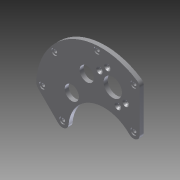
# Autodesk Inventor part: back plate
Saved by Autodesk Inventor 2012 (Build 160160000, 160)
## iProperties
Created: 2012-02-08
Part Number: back plate
Material: Default
Document SubType Name: Modeling
Designer: Antonella Wilby
Density: 1 g/cm^3
Author: Antonella Wilby
Autodesk Inventor part; units mm, degrees
ref_plane "YZ Plane" through (0, 0, 0) normal (1, 0, 0) x (0, 1, 0)
ref_plane "XZ Plane" through (0, 0, 0) normal (0, 1, 0) x (-1, 0, 0)
ref_plane "XY Plane" through (0, 0, 0) normal (0, 0, 1) x (1, 0, 0)
sketch "Sketch1" plane through (0, 0, 0) normal (0, 0, 1) x (1, 0, 0)
  line L0 (-166.2465, 0) -> (95.1399, 0) projected
  line L1 (0, -97.3562) -> (0, 206.312) projected
  circle A0 centre (0, 0) radius 53.975 construction
  arc A1 (39.2886, 39.2886) -> (-55.3511, 4.8426) centre (0, 0) ccw
  line L2 (0, 0) -> (-102.554, 102.554) construction
  circle A2 centre (-50.2894, 50.2894) radius 11.1506
  circle A3 centre (-50.2894, 50.2894) radius 13.335 construction
  circle A4 centre (-50.2894, 50.2894) radius 39.37 construction
  circle A5 centre (-26.9875, 87.3943) radius 11.1506
  circle A6 centre (-26.9875, 87.3943) radius 10.16 construction
  circle A7 centre (-26.9875, 87.3943) radius 33.02 construction
  circle A8 centre (13.589, 89.6653) radius 14.3256
  circle A9 centre (13.589, 89.6653) radius 33.02 construction
  circle A10 centre (0, 0) radius 16.51 construction
  arc A11 (51.2312, 117.4993) -> (-105.7834, 37.5874) centre (-4.3145, 32.4274) ccw
  line L3 (-103.0059, 30.3685) -> (-71.575, -1.0624)
  line L4 (55.5488, 46.0238) -> (55.5488, 109.5238)
  arc A12 (55.5488, 109.5238) -> (51.2312, 117.4993) centre (46.0238, 109.5238) ccw
  arc A13 (-105.7834, 37.5874) -> (-103.0059, 30.3685) centre (-96.2707, 37.1036) ccw
  arc A14 (-71.575, -1.0624) -> (-55.3511, 4.8426) centre (-64.8398, 5.6727) ccw
  arc A15 (39.2886, 39.2886) -> (55.5488, 46.0238) centre (46.0238, 46.0238) ccw
  line L5 (0, 0) -> (46.0238, 46.0238) construction
  line L6 (0, 0) -> (-64.8398, 5.6727) construction
  circle A16 centre (-17.0625, 17.0625) radius 10.16 construction
  point P0 (55.5488, 1.2332)
  point P1 (-51.3036, -21.3339)
  point P2 (55.5488, 114.5184)
  point P3 (-105.911, 33.2736)
  dimension "d0" = 107.95
  dimension "d1" = 45
  dimension "d2" = 1.5875
  dimension "d3" = 22.3012
  dimension "d4" = 26.67
  dimension "d5" = 78.74
  dimension "d6" = 22.3012
  dimension "d7" = 20.32
  dimension "d8" = 66.04
  dimension "d9" = 43.815
  dimension "d10" = 66.04
  dimension "d11" = 28.6512
  dimension "d12" = 33.02
  dimension "d13" = 40.64
  dimension "d43" = 9.525
  dimension "d44" = 9.525
  dimension "d56" = 45
  dimension "d57" = 130
  dimension "d58" = 101.6
  dimension "d59" = 44.45
  dimension "d60" = 63.5
  dimension "d61" = 20.32
  dimension "d63" = 46.99
  dimension "d64" = 26.9875
  dimension "d66" = 13.589
  dimension "d67" = 24.13
  constraints: 17 centre point, 16 point on circle, 10 end point, 8 tangent, 7 coincident, 6 point on line, 2 equal radius, 2 parallel
  measures "d0" diameter of A0
  measures "d1" angle of L1 L2
  measures "d2" radial gap between concentric circles of A1 A0
  measures "d3" diameter of A2
  measures "d4" diameter of A3
  measures "d5" diameter of A4
  measures "d6" diameter of A5
  measures "d7" diameter of A6
  measures "d8" diameter of A7
  measures "d9" distance of A5.centre A2.centre
  measures "d10" diameter of A9
  measures "d11" diameter of A8
  measures "d12" diameter of A10
  measures "d13" distance of A8.centre A5.centre
  measures "d43" radius of A12
  measures "d44" radius of A14
  measures "d56" angle of L5 L0
  measures "d57" angle of L5 L6
  measures "d58" radius of A11
  measures "d59" distance of L3.start L3.end
  measures "d60" distance of L4.start L4.end
  measures "d61" diameter of A16
  measures "d63" distance of A2.centre A16.centre
  measures "d64" distance from line of L1 A5.centre
  measures "d66" distance from line of L1 A8.centre
  measures "d67" distance of A16.centre point (0, 0)
extrude "Base" add sketch "Sketch1" along normal mid plane 6.35 contours L3 A13 A11 L1 A8 A1 A14 L0 | L0 A14 L3 | L1 A8 A11 A12 L4 A15 A1
sketch "Sketch2" plane through (0, 0, 3.175) normal (0, 0, 1) x (1, 0, 0)
  circle A0 centre (13.589, 89.6653) radius 14.3256 projected
  line L0 (-1.0525, 107.1143) -> (27.5194, 73.0637) construction
  line L1 (-7.133, 102.0122) -> (5.028, 112.2165) construction
  line L2 (21.439, 67.9615) -> (33.5999, 78.1658) construction
  line L3 (-166.2465, 0) -> (95.1399, 0) projected
  line L4 (0, -40.0626) -> (0, 196.7631) projected
  dimension "d20" = 44.45
  dimension "d21" = 15.875
  dimension "d73" = 40
  constraints: 6 end point, 4 midpoint, 3 point on line, 2 perpendicular, 1 parallel
  measures "d20" distance of L0.start L0.end
  measures "d21" distance of L1.start L1.end
  measures "d73" angle of L4 L0
hole "Encoder Mount Holes" at (-7.133, 102.0122, 3.175) at (5.028, 112.2165, 3.175) at (21.439, 67.9615, 3.175) at (33.5999, 78.1658, 3.175) direction (0, 0, -1) diameter 5.1054 end through all countersink diameter 9.779 countersink angle 82 clearance for "Flat Head Machine Screw (82)" size "#10" standard "Ansi Unified Screw Threads"
sketch "Sketch4" plane through (0, 0, 3.175) normal (0, 0, 1) x (1, 0, 0)
  arc A0 (55.5488, 109.5238) -> (51.2312, 117.4993) centre (46.0238, 109.5238) ccw projected
  arc A1 (-105.7834, 37.5874) -> (-103.0059, 30.3685) centre (-96.2707, 37.1036) ccw projected
  arc A2 (-71.575, -1.0624) -> (-55.3511, 4.8426) centre (-64.8398, 5.6727) ccw projected
  arc A3 (39.2886, 39.2886) -> (55.5488, 46.0238) centre (46.0238, 46.0238) ccw projected
  arc A4 (39.2886, 39.2886) -> (-55.3511, 4.8426) centre (0, 0) ccw projected
  line L0 (0, 0) -> (-77.2258, 92.0341) construction
  line L1 (0, 0) -> (-11.1042, 126.9216) construction
  line L2 (-166.2465, 0) -> (95.1399, 0) construction
  line L3 (0, -40.0626) -> (0, 196.7631) construction
  dimension "d69" = 5
  dimension "d70" = 40
  dimension "d71" = 120.142
  dimension "d72" = 127.4064
  constraints: 4 coincident, 4 end point
  measures "d69" angle of L3 L1
  measures "d70" angle of L0 L3
  measures "d71" distance of L0.start L0.end
  measures "d72" distance of L0.start L1.end
hole "Standoff Holes" at (-96.2707, 37.1036, 3.175) at (46.0238, 109.5238, 3.175) at (-11.1042, 126.9216, 3.175) at (-77.2258, 92.0341, 3.175) at (-64.8398, 5.6727, 3.175) at (46.0238, 46.0238, 3.175) direction (0, 0, -1) diameter 5.1054 end through all counterbore diameter 9.779 counterbore depth 1.5875 clearance for "Flat Head Machine Screw (82)" size "#10" standard "Ansi Unified Screw Threads"
body "Solid1"
